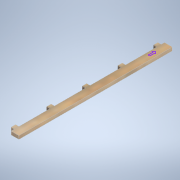
# Autodesk Inventor part: steun
Saved by Autodesk Inventor 2021 (Build 250183000, 183)
## iProperties
Created: 2021-03-16
Part Number: steun
Material: Wood (Maple)
Document SubType Name: Modeling
Designer: ZiweZhang
Density: 0.67 g/cm^3
Appearance: Natural Maple - Glossy Dark Tint
Author: ZiweZhang
Autodesk Inventor part; units mm, degrees
ref_plane "YZ Plane" through (0, 0, 0) normal (1, 0, 0) x (0, 1, 0)
ref_plane "XZ Plane" through (0, 0, 0) normal (0, 1, 0) x (-1, 0, 0)
ref_plane "XY Plane" through (0, 0, 0) normal (0, 0, 1) x (1, 0, 0)
sketch "Sketch1" plane through (0, 0, 0) normal (0, 1, 0) x (-1, 0, 0)
  line L0 (2, -0.85) -> (2, -3.75)
  line L1 (-5, 133.15) -> (2, 133.15)
  line L2 (-5, -3.75) -> (-5, 133.15)
  line L3 (2, -0.85) -> (5, -0.85)
  line L4 (5, -0.85) -> (5, 3.15)
  line L5 (5, 3.15) -> (2, 3.15)
  line L6 (2, 30.9) -> (5, 30.9)
  line L7 (5, 30.9) -> (5, 34.9)
  line L8 (5, 34.9) -> (2, 34.9)
  line L9 (2, 62.65) -> (5, 62.65)
  line L10 (5, 62.65) -> (5, 66.65)
  line L11 (5, 66.65) -> (2, 66.65)
  line L12 (2, 94.4) -> (5, 94.4)
  line L13 (5, 94.4) -> (5, 98.4)
  line L14 (5, 98.4) -> (2, 98.4)
  line L15 (2, 3.15) -> (2, 30.9)
  line L16 (2, 34.9) -> (2, 62.65)
  line L17 (2, 66.65) -> (2, 94.4)
  line L18 (2, 126.15) -> (5, 126.15)
  line L19 (5, 126.15) -> (5, 130.15)
  line L20 (5, 130.15) -> (2, 130.15)
  line L21 (2, 98.4) -> (2, 126.15)
  line L22 (2, -0.85) -> (2, -3.75)
  line L23 (2, -3.75) -> (-5, -3.75)
  line L24 (2, 130.15) -> (2, 133.15)
  point P0 (0, 0)
  point P1 (2, 133.15)
  dimension "d35" = 3
  dimension "d36" = 4
  dimension "d46" = 90
  dimension "d52" = 31.75
  dimension "d57" = 2.9
  constraints: 50 end point, 6 perpendicular, 3 collinear, 2 vertical, 1 horizontal, 27 other
  measures "d35" distance of L0.start L3.end
  measures "d36" distance of L3.end L4.end
  measures "d46" angle of L2 L1
  measures "d52" distance of L3.end L6.end
  measures "d57" distance of L0.end L0.start
extrude "Extrusion1" add sketch "Sketch1" along normal blind 3
sketch "Sketch4" plane through (0, 3, 0) normal (0, 1, 0) x (1, 0, 0)
  line L0 (1.7141, -13.1698) -> (0.2738, -13.1698)
  line L1 (0.2738, -13.1698) -> (0.2738, -8.8733)
  line L2 (0.2738, -8.8733) -> (-0.6051, -8.8733)
  line L3 (-0.6051, -8.8733) -> (0.9939, -7.2743)
  line L4 (0.9939, -7.2743) -> (2.5929, -8.8733)
  line L5 (1.7141, -13.1698) -> (1.7141, -8.8733)
  line L6 (1.7141, -8.8733) -> (2.5929, -8.8733)
  constraints: 14 end point, 4 perpendicular, 1 horizontal, 1 point on line, 1 vertical
body "Solid1"
